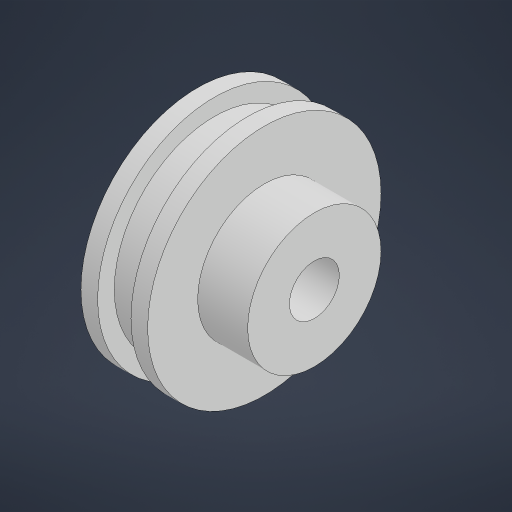
# Autodesk Inventor part: Pulley_OutSide
Saved by Autodesk Inventor 2024.2 (Build 282272000, 272)
## iProperties
Created: 2023-12-22
Part Number: Pulley_OutSide
Material: 一般
Document SubType Name: Modeling
Designer: Hanaoka
Density: 1 g/cm^3
Appearance: 既定
Author: Hanaoka
Autodesk Inventor part; units mm, degrees
ref_plane "YZ Plane" through (0, 0, 0) normal (1, 0, 0) x (0, 1, 0)
ref_plane "XZ Plane" through (0, 0, 0) normal (0, 1, 0) x (-1, 0, 0)
ref_plane "XY Plane" through (0, 0, 0) normal (0, 0, 1) x (1, 0, 0)
sketch "スケッチ1" plane through (0, 0, 0) normal (0, 1, 0) x (-1, 0, 0)
  line L0 (4, 0) -> (4, -7)
  line L1 (4, -7) -> (3, -7)
  line L2 (3, -7) -> (3, -6)
  line L3 (3, -6) -> (1, -6)
  line L4 (1, -6) -> (1, -7)
  line L5 (1, -7) -> (0, -7)
  line L6 (0, -7) -> (0, 0)
  line L7 (4.8, 0) -> (-0.8, 0) projected
  line L8 (4, -1.5) -> (0, -1.5)
  point P0 (1, -6.5)
  dimension "d0" = 1.5
  dimension "d1" = 7
  dimension "d2" = 1
  dimension "d3" = 2
  dimension "d4" = 1
  constraints: 16 end point, 4 point on line, 4 vertical, 3 perpendicular, 1 collinear, 1 horizontal, 1 midpoint
  measures "d0" distance from line of L6.end L8
  measures "d1" distance of L0.start L0.end
  measures "d2" distance of L1.end L2.end
  measures "d3" distance of L2.end L3.end
  measures "d4" distance of L4.end L5.end
revolve "回転1" add sketch "スケッチ1" angle 360 about axis through (-10, 0, 0) along (1, 0, 0) contours L0 L1 L2 L3 L4 L5 L6 L8
sketch "スケッチ2" plane through (0, 0, 0) normal (1, 0, 0) x (0, 0, -1)
  circle A0 centre (0, 0) radius 4
  circle A1 centre (0, 0) radius 1.5 projected
  dimension "d6" = 8
  constraints: 1 centre point, 1 coincident
  measures "d6" diameter of A0
extrude "押し出し1" add sketch "スケッチ2" along normal blind 3
